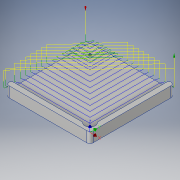
# Autodesk Inventor part: Tastplatte
Saved by Autodesk Inventor 2019 (Build 230136000, 136)
## iProperties
Created: 2021-05-14
Part Number: Tastplatte
Material: Aluminium 6061
Document SubType Name: Modeling
Designer: Michael Sumper
Density: 2.7 g/cm^3
Appearance: Aluminium - flach
Author: Michael Sumper
Autodesk Inventor part; units mm, degrees
ref_plane "YZ Plane" through (0, 0, 0) normal (1, 0, 0) x (0, 1, 0)
ref_plane "XZ Plane" through (0, 0, 0) normal (0, 1, 0) x (-1, 0, 0)
ref_plane "XY Plane" through (0, 0, 0) normal (0, 0, 1) x (1, 0, 0)
sketch "Skizze1" plane through (0, 0, 0) normal (0, 1, 0) x (-1, 0, 0)
  line L0 (-37, 40) -> (37, 40)
  line L1 (40, 37) -> (40, -37)
  line L2 (37, -40) -> (-37, -40)
  line L3 (-40, -37) -> (-40, 37)
  line L4 (-40, 40) -> (40, -40) construction
  line L5 (40, 40) -> (-40, -40) construction
  arc A0 (40, 37) -> (37, 40) centre (37, 37) ccw
  arc A1 (-37, 40) -> (-40, 37) centre (-37, 37) ccw
  arc A2 (-40, -37) -> (-37, -40) centre (-37, -37) ccw
  arc A3 (37, -40) -> (40, -37) centre (37, -37) ccw
  point P0 (0, 0)
  dimension "d0" = 80
  dimension "d1" = 80
  dimension "d2" = 3
  dimension "d3" = 3
  dimension "d4" = 3
  dimension "d5" = 3
  constraints: 12 end point, 8 point on circle, 8 point on line, 8 tangent, 4 centre point, 2 midpoint, 2 parallel, 1 horizontal, 1 perpendicular
  measures "d0" distance of L4.end L5.end
  measures "d1" distance of L5.start L4.end
  measures "d2" radius of A0
  measures "d3" radius of A1
  measures "d4" radius of A2
  measures "d5" radius of A3
extrude "Extrusion1" add sketch "Skizze1" along normal blind 12
sketch "Skizze2" plane through (0, 12, 0) normal (0, 1, 0) x (1, 0, 0)
  line L0 (-40, 37) -> (-40, -37) projected
  arc A0 (-40, -37) -> (-37, -40) centre (-37, -37) ccw projected
  line L1 (-37, -40) -> (37, -40) projected
  arc A1 (37, -40) -> (40, -37) centre (37, -37) ccw projected
  line L2 (40, -37) -> (40, 37) projected
  arc A2 (40, 37) -> (37, 40) centre (37, 37) ccw projected
  line L3 (37, 40) -> (-37, 40) projected
  arc A3 (-37, 40) -> (-40, 37) centre (-37, 37) ccw projected
  line L4 (-35, -35) -> (-35, 35) construction
  line L5 (-35, 35) -> (35, 35) construction
  line L6 (35, 35) -> (35, -28)
  line L7 (28, -35) -> (-35, -35)
  line L8 (-35, -35) -> (-40, -35)
  line L9 (35, 35) -> (35, 40)
  arc A4 (28, -35) -> (35, -28) centre (32, -32) ccw
  point P0 (0, 0)
  dimension "d8" = 5
  dimension "d21" = 10
  constraints: 12 end point, 2 perpendicular, 2 point on circle, 2 point on line, 1 centre point, 1 horizontal, 1 vertical, 2 other
  measures "d8" distance between parallel lines of L0 L4
  measures "d21" diameter of A4
extrude "Extrusion2" cut sketch "Skizze2" against normal blind 6 contours A3 L3 L9 L6 A4 L7 L8 L0
fillet "Rundung1" radius 2 1 edges at (-40, 9, 35)
sketch "Skizze3" plane through (0, 0, 0) normal (0, -1, 0) x (1, 0, 0)
  arc A0 (-40, -37) -> (-37, -40) centre (-37, -37) ccw projected
  line L0 (-37, -37) -> (0, 0) construction
  line L1 (-37, -37) -> (-29.9289, -29.9289) construction
  dimension "d13" = 10
  constraints: 4 end point, 1 coincident, 1 point on line
  measures "d13" distance of L0.start L1.end
hole "Bohrung1" at (-29.9289, 0, -29.9289) direction (0, 1, 0) diameter 2.459 end through all thread size "M3x0.5" class "6H" standard "ISO Metric profile"
sketch "Skizze4" plane through (-37, 0, 40) normal (0, 0, 1) x (1, 0, 0)
  line L0 (-3, 0) -> (0, 0) projected
  line L1 (74, 0) -> (0, 0) projected
  line L2 (74, 0) -> (77, 0) projected
  line L3 (-3, 2) -> (0, 2)
  line L4 (0, 2) -> (74, 2)
  line L5 (74, 2) -> (77, 2)
  line L6 (-3, 0) -> (-3, 6) projected
  line L7 (77, 0) -> (77, 12) projected
  point P0 (37, 0)
  dimension "d22" = 2
  constraints: 6 end point, 2 other
  measures "d22" distance between parallel lines of L1 L4
extrude "Extrusion3" cut sketch "Skizze4" against normal blind 80
